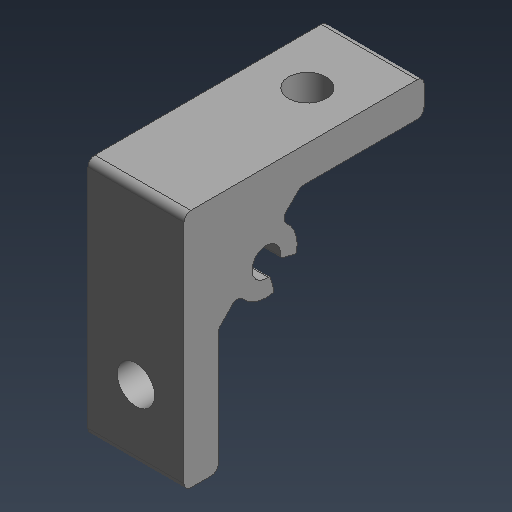
# Autodesk Inventor part: NBLTS5_b
Saved by Autodesk Inventor 2021 (Build 250183000, 183)
## iProperties
Category: PARTsolutions
Company: MISUMI
Part Number: NBLTS5_b
Material: 一般
Catalog Web Link: www.cadenas.de
Description: NBLTS5,HBLTS5,HBLTS5-4,HBLTSB5,HBLTH5,HBLTHB5,HBLTV5,HBLTVB5,HBLTF5,HBLTSW5,HBLTVW5,HBLTD5,HBLTDB5,NBLTT5,HBLTT5,HBLTDW5,HBLTTW5,HBLTVWB5,HBKTS5,HBKTSB5_body-Brackets - 5 Series, Thick Brackets, 1 Slot
Vendor: MISUMI
Document SubType Name: Modeling
Designer: partserver
Manufacturer: MISUMI
Mass: 5.62389 g
Surface Area: 29.9355 cm^2
Volume: 5.62389 cm^3
Density: 1 g/cm^3
Appearance: PSOLRGB-192-192-192
PSOL_IDENT_0: {$CADENAS_DATA\23d-libs\misumi\metric\38_al_extrusions_blackets\5\hblts5.prj},314 {VTYP=3D},{NB=NBLT
PSOL_IDENT_1: S5_b},{LINA=NBLTS5},{NN=NBLTS5,HBLTS5,HBLTS5-4,HBLTSB5,HBLTH5,HBLTHB5,HBLTV5,HBLTVB5,HBLTF5,HBLTSW5,
PSOL_IDENT_2: HBLTVW5,HBLTD5,HBLTDB5,NBLTT5,HBLTT5,HBLTDW5,HBLTTW5,HBLTVWB5,HBKTS5,HBKTSB5_body},{DATE=08.06.2021
PSOL_IDENT_3: 08:24:58},{GEOMDATE=10.10.2017 07:15:23},{VERSION=},{LINEID=70},{WBVAR=ALT1,ALT2},{WBNUMERIC=}  {NB=
PSOL_IDENT_4: NBLTS5_b},{LINA=NBLTS5},{KT=4},{PN=NBLTS5},{TP=NBLTS5},{NOH=1},{NOHV=1},{MAT=JIS-A6063S-T5},{ST=Anod
PSOL_IDENT_5: izing},{TYPE=NBLTS5},{FEAT=Thick Bracket},{ALT1=},{ALT2=},{MASS=15},{AB=CBM5-10},{NOB=2},{AN=HNTT5-5
PSOL_IDENT_6: },{NON=2},{AL=833},{W=14},{H=35},{DP=35},{T=5},{HDIS=0},{DPOS=12},{HH1=25},{HV1=25},{DIA=5.5},{ALT1O
PSOL_IDENT_7: PT='','w/o C (Mounting Holes for Cover','-C','with C (Mounting Holes for Cover)'},{ALT2OPT= '' , 'w/
PSOL_IDENT_8: o Set Applicable Bolt & Nut' , '-SET' , 'with SET (Set Applicable Bolt & Nut)' , '-SST' , 'with SST
PSOL_IDENT_9: (Stainless Steel Set Applicable Bolt & Nut)' , '-SEP' , 'with SEP (Post Assembly Spring Nuts Set App
PSOL_IDENT_10: licable Bolt & Nut)' , '-SSP' , 'with SSP (Post Assembly Spring Nuts, Stainless Steel Set Applicable
PSOL_IDENT_11: Bolt & Nut)'},{R=1},{R1=0.3},{APOSV=17},{VER=2},{PR=4},{M=5},{M1=5}
NB: NBLTS5_b
NN: NBLTS5,HBLTS5,HBLTS5-4,HBLTSB5,HBLTH5,HBLTHB5,HBLTV5,HBLTVB5,HBLTF5,HBLTSW5,HBLTVW5,HBLTD5,HBLTDB5,NBLTT5,HBLTT5,HBLTDW5,HBLTTW5,HBLTVWB5,HBKTS5,HBKTSB5_body
NT: Brackets - 5 Series, Thick Brackets, 1 Slot
NBSYN: $PN._b
LINA: NBLTS5
CATALOG: Misumi
PN: NBLTS5
TP: NBLTS5
MAT: JIS-A6063S-T5
ST: Anodizing
FEAT: Thick Bracket
ALT1: w/o C (Mounting Holes for Cover
ALT2: w/o Set Applicable Bolt & Nut
MASS: 15
AB: CBM5-10
NOB: 2
AN: HNTT5-5
NON: 2
AL: 833
M: 5
M1: 5
SUPPLIER: MISUMI
ARTICLENO: NBLTS5_b
BOMINFO: NBLTS5
CREATOR: CADENAS GmbH
購入先: ミスミ
在庫数: 0.0
Title: NBLTS5
Author: Cadenas PARTsolutions
Comments: Brackets - 5 Series, Thick Brackets, 1 Slot
Autodesk Inventor part; units mm, degrees
sketch "Sketch_1" plane through (0, 0, 0) normal (1, 0, 0) x (0, 1, 0)
  line L0 (4, 35) -> (1, 35)
  arc A0 (1, 35) -> (0, 34) centre (1, 34) ccw
  line L1 (0, 34) -> (0, 1)
  arc A1 (0, 1) -> (1, 0) centre (1, 1) ccw
  line L2 (1, 0) -> (34, 0)
  arc A2 (34, 0) -> (35, 1) centre (34, 1) ccw
  line L3 (35, 1) -> (35, 4)
  arc A3 (35, 4) -> (34, 5) centre (34, 4) ccw
  line L4 (34, 5) -> (17.4142, 5)
  arc A4 (16.7071, 5.2929) -> (17.4142, 5) centre (17.4142, 6) ccw
  line L5 (16.7071, 5.2929) -> (14.878, 7.122)
  arc A5 (14.9333, 8.5874) -> (14.878, 7.122) centre (15.5851, 7.8291) ccw
  arc A6 (14.9333, 8.5874) -> (16.4188, 12.8512) centre (12, 12) ccw
  arc A7 (16.4188, 12.8512) -> (16.0465, 13.0843) centre (16.1242, 12.7945) ccw
  line L6 (16.0465, 13.0843) -> (14.3, 12.6163)
  arc A8 (14.3, 12.6163) -> (14.0805, 12.2857) centre (14.3777, 12.3265) ccw
  arc A9 (12.2857, 14.0805) -> (14.0805, 12.2857) centre (12, 12) ccw
  arc A10 (12.2857, 14.0805) -> (12.6163, 14.3) centre (12.3265, 14.3777) ccw
  line L7 (12.6163, 14.3) -> (13.0843, 16.0465)
  arc A11 (13.0843, 16.0465) -> (12.8512, 16.4188) centre (12.7945, 16.1242) ccw
  arc A12 (12.8512, 16.4188) -> (8.5874, 14.9333) centre (12, 12) ccw
  arc A13 (7.122, 14.878) -> (8.5874, 14.9333) centre (7.8291, 15.5851) ccw
  line L8 (7.122, 14.878) -> (5.2929, 16.7071)
  arc A14 (5, 17.4142) -> (5.2929, 16.7071) centre (6, 17.4142) ccw
  line L9 (5, 17.4142) -> (5, 34)
  arc A15 (5, 34) -> (4, 35) centre (4, 34) ccw
  constraints: 32 point on circle, 20 end point, 16 centre point
extrude "Extrusion1" add sketch "Sketch_1" along normal mid plane 14
sketch "Sketch_2" plane through (0, 0, 0) normal (0, 0, 1) x (1, 0, 0)
  circle A0 centre (0, 25) radius 2.75
  constraints: 1 centre point
extrude "Extrusion2" cut sketch "Sketch_2" along normal mid plane 10
sketch "Sketch_3" plane through (0, 0, 0) normal (0, 1, 0) x (-1, 0, 0)
  circle A0 centre (0, 25) radius 2.75
  constraints: 1 centre point
extrude "Extrusion3" cut sketch "Sketch_3" along normal mid plane 10
ref_plane "bracket_to_dummy_XY" through (0, 0, 0) normal (0, 1, 0) x (1, 0, 0)
ref_plane "bracket_to_dummy_YZ" through (0, 0, 0) normal (1, 0, 0) x (0, 0, -1)
ref_plane "bracket_to_dummy_ZX" through (0, 0, 0) normal (0, 0, -1) x (0, 1, 0)
ref_plane "to_bolt_1_6_XY" through (0, 25, 5) normal (0, 0, 1) x (1, 0, 0)
ref_plane "to_bolt_1_6_YZ" through (0, 25, 5) normal (1, 0, 0) x (0, 1, 0)
ref_plane "to_bolt_1_6_ZX" through (0, 25, 5) normal (0, 1, 0) x (0, 0, 1)
ref_plane "to_bolt_1_6_base_XY" through (0, 5, 25) normal (0, 1, 0) x (1, 0, 0)
ref_plane "to_bolt_1_6_base_YZ" through (0, 5, 25) normal (1, 0, 0) x (0, 0, -1)
ref_plane "to_bolt_1_6_base_ZX" through (0, 5, 25) normal (0, 0, -1) x (0, 1, 0)
ref_plane "to_nut_1_6_XY" through (0, 25, -2) normal (0, 0, 1) x (1, 0, 0)
ref_plane "to_nut_1_6_YZ" through (0, 25, -2) normal (1, 0, 0) x (0, 1, 0)
ref_plane "to_nut_1_6_ZX" through (0, 25, -2) normal (0, 1, 0) x (0, 0, 1)
ref_plane "to_nut_1_6_base_XY" through (0, -2, 25) normal (0, 1, 0) x (1, 0, 0)
ref_plane "to_nut_1_6_base_YZ" through (0, -2, 25) normal (1, 0, 0) x (0, 0, -1)
ref_plane "to_nut_1_6_base_ZX" through (0, -2, 25) normal (0, 0, -1) x (0, 1, 0)
ref_plane "to_screw_XY" through (0, 5, 25) normal (0, 1, 0) x (1, 0, 0)
ref_plane "to_screw_YZ" through (0, 5, 25) normal (1, 0, 0) x (0, 0, -1)
ref_plane "to_screw_ZX" through (0, 5, 25) normal (0, 0, -1) x (0, 1, 0)
ref_plane "to_screw10_XY" through (0, 5, 25) normal (0, 1, 0) x (1, 0, 0)
ref_plane "to_screw10_YZ" through (0, 5, 25) normal (1, 0, 0) x (0, 0, -1)
ref_plane "to_screw10_ZX" through (0, 5, 25) normal (0, 0, -1) x (0, 1, 0)
ref_plane "to_screw2_XY" through (0, 5, 25) normal (0, 1, 0) x (1, 0, 0)
ref_plane "to_screw2_YZ" through (0, 5, 25) normal (1, 0, 0) x (0, 0, -1)
ref_plane "to_screw2_ZX" through (0, 5, 25) normal (0, 0, -1) x (0, 1, 0)
ref_plane "to_screw3_XY" through (0, 25, 5) normal (0, 0, 1) x (1, 0, 0)
ref_plane "to_screw3_YZ" through (0, 25, 5) normal (1, 0, 0) x (0, 1, 0)
ref_plane "to_screw3_ZX" through (0, 25, 5) normal (0, 1, 0) x (0, 0, 1)
ref_plane "to_screw4_XY" through (0, 25, 5) normal (0, 0, 1) x (1, 0, 0)
ref_plane "to_screw4_YZ" through (0, 25, 5) normal (1, 0, 0) x (0, 1, 0)
ref_plane "to_screw4_ZX" through (0, 25, 5) normal (0, 1, 0) x (0, 0, 1)
ref_plane "to_screw5_XY" through (0, 5, 25) normal (0, 1, 0) x (1, 0, 0)
ref_plane "to_screw5_YZ" through (0, 5, 25) normal (1, 0, 0) x (0, 0, -1)
ref_plane "to_screw5_ZX" through (0, 5, 25) normal (0, 0, -1) x (0, 1, 0)
ref_plane "to_screw6_XY" through (0, 5, 25) normal (0, 1, 0) x (1, 0, 0)
ref_plane "to_screw6_YZ" through (0, 5, 25) normal (1, 0, 0) x (0, 0, -1)
ref_plane "to_screw6_ZX" through (0, 5, 25) normal (0, 0, -1) x (0, 1, 0)
ref_plane "to_screw7_XY" through (0, 25, 5) normal (0, 0, 1) x (1, 0, 0)
ref_plane "to_screw7_YZ" through (0, 25, 5) normal (1, 0, 0) x (0, 1, 0)
ref_plane "to_screw7_ZX" through (0, 25, 5) normal (0, 1, 0) x (0, 0, 1)
ref_plane "to_screw8_XY" through (0, 25, 5) normal (0, 0, 1) x (1, 0, 0)
ref_plane "to_screw8_YZ" through (0, 25, 5) normal (1, 0, 0) x (0, 1, 0)
ref_plane "to_screw8_ZX" through (0, 25, 5) normal (0, 1, 0) x (0, 0, 1)
ref_plane "to_screw9_XY" through (0, 25, 5) normal (0, 0, 1) x (1, 0, 0)
ref_plane "to_screw9_YZ" through (0, 25, 5) normal (1, 0, 0) x (0, 1, 0)
ref_plane "to_screw9_ZX" through (0, 25, 5) normal (0, 1, 0) x (0, 0, 1)
body "Solid1"
